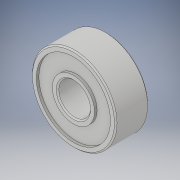
# Autodesk Inventor part: Homemade_bearing
Saved by Autodesk Inventor 2018 (Build 220112000, 112)
## iProperties
Created: 2018-07-13
Part Number: Homemade_bearing
Material: Generic
Document SubType Name: Modeling
Designer: baoan
Density: 1 g/cm^3
Appearance: Default
Author: baoan
Autodesk Inventor part; units mm, degrees
ref_plane "YZ Plane" through (0, 0, 0) normal (1, 0, 0) x (0, 1, 0)
ref_plane "XZ Plane" through (0, 0, 0) normal (0, 1, 0) x (-1, 0, 0)
ref_plane "XY Plane" through (0, 0, 0) normal (0, 0, 1) x (1, 0, 0)
sketch "Sketch1" plane through (0, 0, 0) normal (0, 0, 1) x (1, 0, 0)
  circle A0 centre (0, 0) radius 2.3813
  circle A1 centre (0, 0) radius 6.35
  dimension "d0" = 4.7625
  dimension "d1" = 12.7
  constraints: 2 centre point, 2 coincident
  measures "d0" diameter of A0
  measures "d1" diameter of A1
extrude "Extrusion1" add sketch "Sketch1" along normal mid plane 4.9784
chamfer "Chamfer1" distance 0.1984 angle 45 4 edges at (-6.35, 0, 2.4892) (-2.3813, 0, 2.4892) (-6.35, 0, -2.4892) (-2.3813, 0, -2.4892)
sketch "Sketch2" plane through (0, 0, 0) normal (0, 1, 0) x (-1, 0, 0)
  line L0 (-6.1516, 2.4892) -> (6.1516, 2.4892) projected
  line L1 (2.5797, 2.4892) -> (-2.5797, 2.4892) projected
  line L2 (-5.5626, 2.4892) -> (-3.1686, 2.4892)
  line L3 (-3.1686, 2.4892) -> (-3.1686, 2.1082)
  line L4 (-3.1686, 2.1082) -> (-5.5626, 2.1082)
  line L5 (-5.5626, 2.1082) -> (-5.5626, 2.4892)
  line L6 (-6.35, -2.2908) -> (-6.35, 2.2908) projected
  line L7 (-2.3813, -2.2908) -> (-2.3813, 2.2908) projected
  line L8 (0, 0) -> (0, 3.7082)
  dimension "d7" = 0.381
  dimension "d8" = 0.7874
  dimension "d9" = 0.7874
  constraints: 10 end point, 2 parallel, 1 horizontal, 1 perpendicular, 1 point on line, 1 vertical
  measures "d7" distance of L4.end L2.start
  measures "d8" distance between parallel lines of L6 L5
  measures "d9" distance between parallel lines of L7 L3
revolve "Revolution1" cut sketch "Sketch2" angle 360 about axis through (0, 0, 0) along (0, 0, 1)
mirror "Mirror1" about plane through (0, 0, 0) normal (0, 0, 1) of "Revolution1"
equation "\"d9\" = d8"
body "Solid1"
